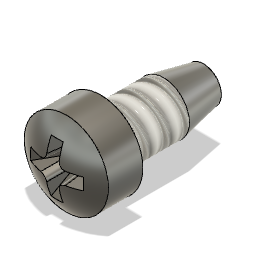
assembly (Autodesk Fusion 360 archive; units mm, degrees)
design "Type II Cross Recessed Fillister Head Tapping Screw ANSI B18.6.4 5-20 x 0.25 Type BF Steel Grade 2 Plain"
description: Type II Cross Recessed Fillister Head Tapping Screw ANSI B18.6.4 5-20 x 0.25 Type BF
Autodesk Fusion 360 part; units mm, degrees
sketch "Sketch1" plane through (0, 0, 0) normal (0, 1, 0) x (1, 0, 0)
  line L0 (-1.5875, 0) -> (-1.5875, 6.35)
  line L1 (-1.5875, 6.35) -> (0, 6.35)
  line L2 (0, 6.35) -> (0, -3.048)
  line L3 (-1.5875, 0) -> (-2.6035, 0)
  line L4 (-2.6035, 0) -> (-2.6035, -2.1342)
  arc A0 (-2.6035, -2.1342) -> (0, -3.048) centre (0, 1.1176) ccw
  dimension "d9" = 3.175
  dimension "d66" = 5.207
  dimension "d67" = 3.048
  dimension "d68" = 6.35
  dimension "d70" = 4.1656
  constraint perpendicular L0 L1
  constraint perpendicular L0 L3
  constraint coincident origin L3
  constraint vertical L0
  constraint vertical L2
  constraint coincident L2 A0.centre
  constraint perpendicular L3 L4
  constraint coincident origin L2
  measures "d67" vertical distance of L2.end L3.end
  measures "d68" distance of origin L1.end
  measures "d70" radius of A0
revolve "Revolve1" add sketch "Sketch1" angle 360 about axis through (0, 0, -6.35) along (0, 0, 1)
ref_plane "WorkPlane1" through (0, 0, 3.048) normal (0, 0, 1) x (1, 0, 0)
sketch "Sketch2" plane through (0, 0, 3.048) normal (0, 0, 1) x (1, 0, 0)
  circle A0 centre (0, 0) radius 3
  line L0 (-0.3937, 1.8669) -> (-0.3937, 0.3937)
  line L1 (-0.3937, 0.3937) -> (-1.8669, 0.3937)
  line L2 (0, 0) -> (0, 1.8669) construction
  line L3 (0.3937, 0.3937) -> (1.8669, 0.3937)
  line L4 (0.3937, 1.8669) -> (0.3937, 0.3937)
  line L5 (0.3937, -0.3937) -> (1.8669, -0.3937)
  line L6 (0.3937, -1.8669) -> (0.3937, -0.3937)
  line L7 (-0.3937, -1.8669) -> (-0.3937, -0.3937)
  line L8 (-0.3937, -0.3937) -> (-1.8669, -0.3937)
  line L9 (-0.3937, 1.8669) -> (0.3937, 1.8669)
  line L10 (-1.8669, 0.3937) -> (-1.8669, -0.3937)
  line L11 (-0.3937, -1.8669) -> (0.3937, -1.8669)
  line L12 (1.8669, -0.3937) -> (1.8669, 0.3937)
  line L13 (1.75, 0) -> (22.5, 0)
  circle A1 centre (0, 0) radius 1.5
  dimension "d22" = 0.7874
  dimension "d57" = 3.7338
  constraint perpendicular L0 L1
  constraint coincident A0.centre L2.start
  constraint symmetric L0.start L2 L4.start
  constraint symmetric L0.end L2 L3.start
  constraint symmetric L1.end L2 L3.end
  constraint perpendicular L4 L9
  constraint perpendicular L8 L10
  constraint equal L9 L10
  constraint equal L0 L1
  constraint symmetric L1 L8 L13
  constraint horizontal L0.start L2.end
  constraint vertical L2
  constraint symmetric L3 L5 L13
  constraint symmetric L9 L11 L13
  constraint collinear L4 L6
  measures "d22" horizontal distance of L0.start L4.start
  measures "d57" distance of L10 L12
extrude "Extrude1" cut sketch "Sketch2" against normal blind 2.0066 draft -4 contours L0 L4 L9 A1 | L0 L1 L3 L4 L5 L6 L7 L8 A1 | L1 L8 L10 A1 | L3 L5 L12 A1 | L6 L7 L11 A1
fillet "Fillet3" radius 0.3734 4 edges at (-0.3223, 0.3223, 2.0263) (0.3223, 0.3223, 2.0263) (0.3223, -0.3223, 2.0263) (-0.3223, -0.3223, 2.0263)
draft "Draft1" angle 30 neutral plane through (0, 0, 3.048) pull (0, 0, 1) 4 faces at (1.7634, 0.0403, 1.5673) (-0.0403, 1.7634, 1.5673) (-1.7634, 0, 1.5679) (0.0403, -1.7634, 1.5673)
thread "Thread1" "Inch Tapping Threads 0.125 5-20 2B" major diameter 3.2131 minor diameter 2.3368 pitch 1.27 angle 60 resizes the face on face at (0.2507, 1.5676, -3.1814)
sketch "Sketch5" plane through (0, 0, 0) normal (0, 1, 0) x (1, 0, 0)
  line L0 (-1.6193, 3.81) -> (-1.1049, 6.35)
  line L1 (-1.6193, 3.81) -> (-1.6192, 6.35)
  line L2 (0, 6.35) -> (0, -3.048)
  line L3 (-1.6192, 6.35) -> (0, 6.35)
  dimension "d100" = 2.54
  dimension "d101" = 1.1049
  dimension "d102" = 1.6193
  constraint coincident L2.start L3.end
  constraint perpendicular L1 L3
  constraint coincident L0.end L3
  constraint perpendicular L2 L3
  measures "d100" vertical distance of L0.start L0.end
  measures "d101" horizontal distance of origin L0.end
  measures "d102" horizontal distance of origin L0.start
revolve "Revolve2" cut sketch "Sketch5" angle 360 about axis through (0, 0, -6.35) along (0, 0, 1)
equation "d9 = adsk_nomdia"
equation "d22 = adsk_philwidth"
equation "d31 = -adsk_phildepth"
equation "d57 = adsk_phildia"
equation "d59 = adsk_phildia * 0.1"
equation "d66 = adsk_headdia"
equation "d67 = adsk_headh"
equation "d68 = adsk_nomlen"
equation "d70 = adsk_headdia * 0.8"
equation "d71 = adsk_headh"
equation "adsk_nomlen = 0.25 in"
equation "adsk_headh = 0.12 in"
equation "adsk_headdia = 0.205 in"
equation "adsk_nomdia = 0.125 in"
equation "adsk_phildia = 0.147 in"
equation "adsk_philwidth = 0.031 in"
equation "adsk_phildepth = 0.079 in"
equation "adsk_startlen = 0.10 in"
equation "adsk_endpointdia = 0.087 in"
equation "d100 = adsk_startlen"
equation "d101 = adsk_endpointdia / 2"
equation "d102 = adsk_nomdia * 0.51"
